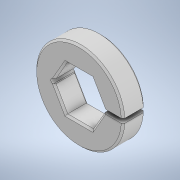
# Autodesk Inventor part: Hex Shaft Collar
Saved by Autodesk Inventor 2020 (Build 240168000, 168)
## iProperties
Created: 2020-01-16
Part Number: Hex Shaft Collar
Material: Generic
Document SubType Name: Modeling
Designer: aidan
Density: 1 g/cm^3
Appearance: Default
Author: aidan
Autodesk Inventor part; units mm, degrees
ref_plane "YZ Plane" through (0, 0, 0) normal (1, 0, 0) x (0, 1, 0)
ref_plane "XZ Plane" through (0, 0, 0) normal (0, 1, 0) x (-1, 0, 0)
ref_plane "XY Plane" through (0, 0, 0) normal (0, 0, 1) x (1, 0, 0)
sketch "Sketch1" plane through (0, 0, 0) normal (0, 0, 1) x (1, 0, 0)
  line L0 (-4.3488, 6.4416) -> (3.1302, 6.4416)
  line L1 (3.1302, 6.4416) -> (6.503, 0.5996)
  line L2 (6.503, -0.6704) -> (3.1302, -6.5124)
  line L3 (3.1302, -6.5124) -> (-4.3488, -6.5124)
  line L4 (-4.3488, -6.5124) -> (-7.7708, -0.5853)
  line L5 (-7.7708, 0.5145) -> (-4.3488, 6.4416)
  arc A0 (12.0748, 0.5996) -> (12.0748, -0.6704) centre (-0.6093, -0.0354) ccw
  arc A1 (-8.0883, 0.5996) -> (-8.0883, -0.6704) centre (-8.0883, -0.0354) ccw
  line L6 (-8.0883, 0.5996) -> (-7.7217, 0.5996)
  line L7 (6.503, 0.5996) -> (12.0748, 0.5996)
  line L8 (-8.0883, -0.6704) -> (-7.7217, -0.6704)
  line L9 (6.503, -0.6704) -> (12.0748, -0.6704)
  point P0 (-0.6093, 6.4416)
  dimension "d2" = 12.954
  dimension "d3" = 25.4
  dimension "d4" = 1.27
  constraints: 20 end point, 5 horizontal, 4 point on circle, 4 tangent, 2 centre point, 2 point on line, 1 coincident, 1 midpoint, 9 other
  measures "d2" distance between parallel lines of L3 L0
  measures "d3" diameter of A0
  measures "d4" diameter of A1
extrude "Extrusion1" add sketch "Sketch1" along normal blind 6.35
chamfer "Chamfer1" distance 0.508 angle 45 2 edges at (-13.3093, -0.0354, 6.35) (-13.3093, -0.0354, 0)
chamfer "Chamfer2" distance 0.508 angle 45 12 edges at (-6.0353, 3.5206, 6.35) (-0.6093, 6.4416, 6.35) (4.8166, 3.5206, 6.35) (4.8166, -3.5914, 6.35) (-0.6093, -6.5124, 6.35) (-6.0353, -3.5914, 6.35) (-6.0353, -3.5914, 0) (-6.0353, 3.5206, 0) (-0.6093, -6.5124, 0) (4.8166, -3.5914, 0) (4.8166, 3.5206, 0) (-0.6093, 6.4416, 0)
body "Solid1"
